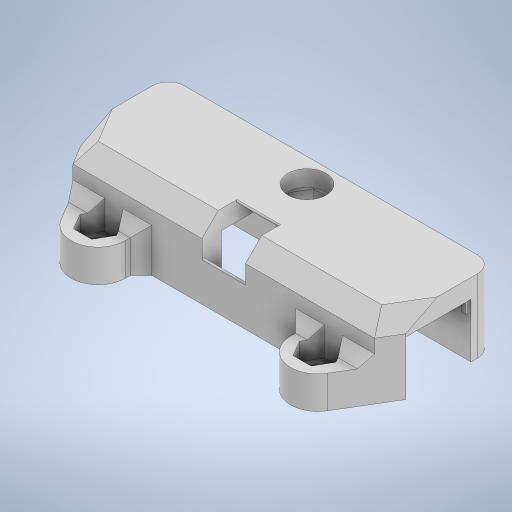
# Autodesk Inventor part: uchwyt_silnikow
Saved by Autodesk Inventor 2023 (Build 270158000, 158)
## iProperties
Created: 2023-08-17
Part Number: uchwyt_silnikow
Material: Ogólny
Document SubType Name: Modeling
Designer: Kamil
Density: 1 g/cm^3
Appearance: Domyślna
Author: Kamil
Autodesk Inventor part; units mm, degrees
ref_plane "YZ Plane" through (0, 0, 0) normal (1, 0, 0) x (0, 1, 0)
ref_plane "XZ Plane" through (0, 0, 0) normal (0, 1, 0) x (-1, 0, 0)
ref_plane "XY Plane" through (0, 0, 0) normal (0, 0, 1) x (1, 0, 0)
sketch "Szkic1" plane through (0, 0, 0) normal (0, 1, 0) x (-1, 0, 0)
  circle A0 centre (-9.75, 6.5) radius 1.75
  circle A1 centre (-50.25, 6.5) radius 1.75
  arc A2 (-31.4825, -12) -> (-28.5175, -12) centre (-30, -11.7713) ccw
  arc A3 (-28.5175, -12) -> (-31.4825, -12) centre (-30, -11.7713) ccw
  arc A4 (-3, -16.2) -> (0, -13.2) centre (-3, -13.2) ccw
  line L0 (0, -12) -> (0, -13.2)
  line L1 (-25.5772, -12) -> (0, -12)
  line L2 (-28.5175, -12) -> (-25.5772, -12)
  arc A5 (-31.4825, -12) -> (-28.5175, -12) centre (-30, -11.7713) ccw
  line L3 (-31.4825, -12) -> (-34.4228, -12)
  line L4 (-34.4228, -12) -> (-60, -12)
  line L5 (-60, -12) -> (-60, -13.2)
  arc A6 (-60, -13.2) -> (-57, -16.2) centre (-57, -13.2) ccw
  line L6 (-3, -16.2) -> (-57, -16.2)
  circle A7 centre (-50.25, 6.5) radius 1.75
  line L7 (-24.852, 0) -> (0, 0)
  line L8 (-35.148, 0) -> (-60, 0)
  circle A8 centre (-9.75, 6.5) radius 1.75
  circle A9 centre (-50.25, 6.5) radius 5
  circle A10 centre (-9.75, 6.5) radius 5
  line L9 (-60, 0) -> (-54.5335, 9.0791)
  line L10 (0, 0) -> (-5.4665, 9.0791)
  line L11 (-14.75, 6.5) -> (-14.75, 0)
  line L12 (-45.25, 6.5) -> (-45.25, 0)
  arc A11 (-27.6792, -16.2) -> (-32.3208, -16.2) centre (-30, -11.7713) ccw
  point P0 (-25.0052, -12)
  point P1 (-34.9948, -12)
  dimension "d0" = 10
  dimension "d1" = 10
  dimension "d2" = 10
  constraints: 26 end point, 16 point on circle, 12 centre point, 6 horizontal, 4 point on line, 4 tangent, 3 coincident, 1 perpendicular, 1 vertical, 4 other
  measures "d0" diameter of A9
  measures "d1" diameter of A10
  measures "d2" diameter of A11
extrude "Wyciągnięcie proste1" add sketch "Szkic1" along normal blind 10 contours L3 L4 A11 L1 L2 A3 | A2 L2 L1 A11 L6 L4 L3 | A11 L6 A6 L5 L4 | L1 L0 A4 L6 A11 | L11 A10 L10 L7 | A10 | L8 L9 A9 L12 | A9
sketch "Szkic2" plane through (0, 10, 0) normal (0, 1, 0) x (1, 0, 0)
  line L0 (57, 16.2) -> (3, 16.2) projected
  arc A0 (3, 16.2) -> (0, 13.2) centre (3, 13.2) ccw projected
  line L1 (0, 13.2) -> (0, 12) projected
  line L2 (0, 12) -> (25.0052, 12) projected
  arc A1 (25.0052, 12) -> (34.9948, 12) centre (30, 11.7713) ccw projected
  line L3 (34.9948, 12) -> (60, 12) projected
  line L4 (60, 12) -> (60, 13.2) projected
  arc A2 (60, 13.2) -> (57, 16.2) centre (57, 13.2) ccw projected
  circle A3 centre (30, 11.7713) radius 1.5 projected
  line L5 (14.75, 0) -> (0, 0) projected
  line L6 (0, 0) -> (5.4665, -9.0791) projected
  arc A4 (5.4665, -9.0791) -> (14.75, -6.5) centre (9.75, -6.5) ccw projected
  line L7 (14.75, -6.5) -> (14.75, 0) projected
  circle A5 centre (9.75, -6.5) radius 1.75 projected
  arc A6 (45.25, -6.5) -> (54.5335, -9.0791) centre (50.25, -6.5) ccw projected
  line L8 (54.5335, -9.0791) -> (60, 0) projected
  line L9 (60, 0) -> (45.25, 0) projected
  line L10 (45.25, 0) -> (45.25, -6.5) projected
  circle A7 centre (50.25, -6.5) radius 1.75 projected
  line L11 (0, 0) -> (60, 0)
  line L12 (60, 0) -> (60, 12)
  line L13 (60, 12) -> (0, 12)
  line L14 (0, 12) -> (0, 0)
  constraints: 8 end point, 2 parallel, 1 horizontal, 1 perpendicular
extrude "Wyciągnięcie proste2" add sketch "Szkic2" along normal blind 3.5 contours A2 L4 L3 L13 A3 L2 L1 A0 L0 | L12 L9 L11 L5 L14 L2 A1 L3 | A1 L13 A3 | L8 A6 L10 L9 | L5 L7 A4 L6
sketch "Szkic3" plane through (0, 0, 0) normal (0, -1, 0) x (1, 0, 0)
  line L0 (14.75, 0) -> (0, 0) projected
  line L1 (14.75, 6.5) -> (14.75, 0) projected
  arc A0 (14.75, 6.5) -> (5.4665, 9.0791) centre (9.75, 6.5) ccw projected
  line L2 (0, 0) -> (5.4665, 9.0791) projected
  circle A1 centre (9.75, 6.5) radius 1.75 projected
  arc A2 (54.5335, 9.0791) -> (45.25, 6.5) centre (50.25, 6.5) ccw projected
  line L3 (45.25, 0) -> (45.25, 6.5) projected
  line L4 (60, 0) -> (45.25, 0) projected
  line L5 (54.5335, 9.0791) -> (60, 0) projected
  circle A3 centre (50.25, 6.5) radius 1.75 projected
  line L6 (14.75, 0) -> (45.25, 0) projected
  line L7 (45.25, 0) -> (14.75, 0)
  line L8 (14.75, 0) -> (14.75, 4)
  line L9 (14.75, 4) -> (45.25, 4)
  line L10 (45.25, 4) -> (45.25, 0)
  dimension "d7" = 4
  constraints: 8 end point, 2 parallel, 1 horizontal, 1 perpendicular, 1 point on line
  measures "d7" distance of L7.end L8.end
extrude "Wyciągnięcie proste3" add sketch "Szkic3" against normal up to surface (13.5 mm away) contours L1 L9 L3 L6
sketch "Szkic4" plane through (0, 13.5, 0) normal (0, 1, 0) x (1, 0, 0)
  circle A0 centre (9.75, -6.5) radius 1.75 projected
  circle A1 centre (50.25, -6.5) radius 1.75 projected
  circle A2 centre (9.75, -6.5) radius 2.9
  circle A3 centre (50.25, -6.5) radius 2.9
  line L0 (11.4243, -3.6) -> (13.0986, -6.5)
  line L1 (13.0986, -6.5) -> (11.4243, -9.4)
  line L2 (11.4243, -9.4) -> (8.0757, -9.4)
  line L3 (8.0757, -9.4) -> (6.4014, -6.5)
  line L4 (6.4014, -6.5) -> (8.0757, -3.6)
  line L5 (8.0757, -3.6) -> (11.4243, -3.6)
  line L6 (51.9243, -3.6) -> (53.5986, -6.5)
  line L7 (53.5986, -6.5) -> (51.9243, -9.4)
  line L8 (51.9243, -9.4) -> (48.5757, -9.4)
  line L9 (48.5757, -9.4) -> (46.9014, -6.5)
  line L10 (46.9014, -6.5) -> (48.5757, -3.6)
  line L11 (48.5757, -3.6) -> (51.9243, -3.6)
  line L12 (0, 0) -> (5.4665, -9.0791) projected
  line L13 (2.1676, -3.6) -> (57.8324, -3.6)
  line L14 (54.5335, -9.0791) -> (60, 0) projected
  arc A4 (60, 13.2) -> (57, 16.2) centre (57, 13.2) ccw projected
  line L15 (57, 16.2) -> (3, 16.2) projected
  arc A5 (3, 16.2) -> (0, 13.2) centre (3, 13.2) ccw projected
  line L16 (0, 13.2) -> (0, 0) projected
  line L17 (0, 0) -> (5.4665, -9.0791) projected
  arc A6 (5.4665, -9.0791) -> (14.75, -6.5) centre (9.75, -6.5) ccw projected
  line L18 (14.75, -6.5) -> (14.75, -4) projected
  line L19 (45.25, -4) -> (14.75, -4) projected
  line L20 (45.25, -4) -> (45.25, -6.5) projected
  arc A7 (45.25, -6.5) -> (54.5335, -9.0791) centre (50.25, -6.5) ccw projected
  line L21 (54.5335, -9.0791) -> (60, 0) projected
  line L22 (60, 0) -> (60, 13.2) projected
  circle A8 centre (9.75, -6.5) radius 1.75 projected
  circle A9 centre (50.25, -6.5) radius 1.75 projected
  circle A10 centre (30, 11.7713) radius 1.5 projected
  point P0 (9.75, -3.6)
  point P1 (50.25, -3.6)
  dimension "d10" = 5.8
  dimension "d11" = 5.8
  constraints: 26 end point, 4 coincident, 3 point on line, 2 midpoint, 2 vertical alignment, 1 horizontal, 30 other
extrude "Wyciągnięcie proste4" cut sketch "Szkic4" against normal blind 7.5 contours L0 L13 L10 L9 L8 L7 L6 L14 A7 L20 L19 L18 A6 L12 L4 L3 L2 L1
extrude "Wyciągnięcie proste5" cut sketch "Szkic4" against normal blind 10.8 contours A0 | A1 | A2 | A2 L0 L1 | A2 L5 L0 | L1 L2 A2 | A2 L4 L5 | L2 L3 A2 | A2 L3 L4 | L11 A3 L10 | A3 | A3 L9 L10 | L11 L6 A3 | A3 L8 L9 | L6 L7 A3 | A3 L7 L8
sketch "Szkic5" plane through (0, 6, 0) normal (0, 1, 0) x (1, 0, 0)
  line L0 (14.75, -4) -> (14.75, -6.5) projected
  line L1 (45.25, -4) -> (14.75, -4) projected
  line L2 (45.25, -6.5) -> (45.25, -4) projected
  arc A0 (45.25, -6.5) -> (54.5335, -9.0791) centre (50.25, -6.5) ccw projected
  line L3 (57.8324, -3.6) -> (54.5335, -9.0791) projected
  line L4 (51.9243, -3.6) -> (57.8324, -3.6) projected
  line L5 (53.5986, -6.5) -> (51.9243, -3.6) projected
  line L6 (51.9243, -9.4) -> (53.5986, -6.5) projected
  line L7 (48.5757, -9.4) -> (51.9243, -9.4) projected
  line L8 (46.9014, -6.5) -> (48.5757, -9.4) projected
  line L9 (48.5757, -3.6) -> (46.9014, -6.5) projected
  line L10 (11.4243, -3.6) -> (48.5757, -3.6) projected
  line L11 (13.0986, -6.5) -> (11.4243, -3.6) projected
  line L12 (11.4243, -9.4) -> (13.0986, -6.5) projected
  line L13 (8.0757, -9.4) -> (11.4243, -9.4) projected
  line L14 (6.4014, -6.5) -> (8.0757, -9.4) projected
  line L15 (8.0757, -3.6) -> (6.4014, -6.5) projected
  line L16 (2.1676, -3.6) -> (8.0757, -3.6) projected
  line L17 (5.4665, -9.0791) -> (2.1676, -3.6) projected
  arc A1 (5.4665, -9.0791) -> (14.75, -6.5) centre (9.75, -6.5) ccw projected
  line L18 (14.75, -4) -> (14.75, -3.6)
  line L19 (45.25, -4) -> (45.25, -3.6)
  point P0 (0, 0)
  constraints: 4 end point, 2 perpendicular, 2 point on line
extrude "Wyciągnięcie proste6" cut sketch "Szkic5" against normal through all contours L18 L10 L19 L1
sketch "Szkic6" plane through (0, 13.5, 0) normal (0, 1, 0) x (1, 0, 0)
  circle A0 centre (30, 11.7713) radius 1.5 projected
  circle A1 centre (30, 11.7713) radius 2.9
  circle A2 centre (30, 11.7713) radius 1.5 projected
  line L0 (31.6743, 14.6713) -> (33.3486, 11.7713)
  line L1 (33.3486, 11.7713) -> (31.6743, 8.8713)
  line L2 (31.6743, 8.8713) -> (28.3257, 8.8713)
  line L3 (28.3257, 8.8713) -> (26.6514, 11.7713)
  line L4 (26.6514, 11.7713) -> (28.3257, 14.6713)
  line L5 (28.3257, 14.6713) -> (31.6743, 14.6713)
  circle A3 centre (30, 11.7713) radius 3.5
  point P0 (0, 0)
  point P1 (30, 14.6713)
  dimension "d20" = 5.8
  dimension "d21" = 7
  constraints: 12 end point, 3 coincident, 1 centre point, 1 midpoint, 1 vertical alignment, 15 other
  measures "d21" diameter of A3
extrude "Wyciągnięcie proste7" cut sketch "Szkic6" against normal blind 3 contours A0 | A1 | A1 L0 L1 | A1 L5 L0 | L1 L2 A1 | A1 L4 L5 | L2 L3 A1 | A1 L3 L4 | A3
extrude "Wyciągnięcie proste8" cut sketch "Szkic6" against normal blind 6 contours A0 | A1 | A1 L0 L1 | A1 L5 L0 | L1 L2 A1 | A1 L4 L5 | L2 L3 A1 | A1 L3 L4
sketch "Szkic7" plane through (0, 10, 0) normal (0, -1, 0) x (1, 0, 0)
  line L0 (60, 0) -> (0, 0) projected
  line L1 (0, -12) -> (0, 0) projected
  line L2 (0, -12) -> (25.0052, -12) projected
  arc A0 (34.9948, -12) -> (25.0052, -12) centre (30, -11.7713) ccw projected
  line L3 (34.9948, -12) -> (60, -12) projected
  line L4 (60, 0) -> (60, -12) projected
  line L5 (34.9948, -12) -> (60, -12) projected
  line L6 (59.4, -12) -> (58.7, -12)
  line L7 (58.7, -12) -> (58.7, -9)
  line L8 (58.7, -9) -> (59.4, -9)
  line L9 (59.4, -9) -> (59.4, -12)
  line L10 (53.6, -12) -> (51.6, -12)
  line L11 (51.6, -12) -> (51.6, -9)
  line L12 (51.6, -9) -> (53.6, -9)
  line L13 (53.6, -9) -> (53.6, -12)
  circle A1 centre (30, -11.7713) radius 1.5 projected
  line L14 (30, -11.7713) -> (30, 0)
  line L15 (60, 0) -> (0, 0) projected
  line L16 (1.3, -12) -> (1.3, -9)
  line L17 (1.3, -9) -> (0.6, -9)
  line L18 (0.6, -9) -> (0.6, -12)
  line L19 (8.4, -12) -> (8.4, -9)
  line L20 (8.4, -9) -> (6.4, -9)
  line L21 (6.4, -9) -> (6.4, -12)
  point P0 (58.7, -10.5)
  point P1 (53.6, -10.5)
  dimension "d26" = 0.7
  dimension "d27" = 3
  dimension "d28" = 0.6
  dimension "d29" = 2
  dimension "d30" = 5.1
  dimension "d31" = 3
  constraints: 30 end point, 8 symmetric about line, 4 parallel, 3 midpoint, 2 horizontal, 2 perpendicular, 2 point on line
  measures "d26" distance of L7.end L8.end
  measures "d27" distance of L6.end L7.end
  measures "d28" distance between parallel lines of L4 L9
  measures "d29" distance of L11.end L12.end
  measures "d30" distance of point (58.7, -10.5) point (53.6, -10.5)
  measures "d31" distance of L10.end L11.end
extrude "Wyciągnięcie proste9" add sketch "Szkic7" along normal blind 0.4 contours L3 L7 L8 L9 | L18 L17 L16 L2 | L11 L12 L13 L3 | L2 L21 L20 L19
sketch "Szkic8" plane through (34.9948, 0, -12) normal (0, 0, 1) x (1, 0, 0)
  line L0 (-33.6948, 9.6) -> (-34.3948, 9.6) projected
  line L1 (-26.5948, 9.6) -> (-28.5948, 9.6) projected
  line L2 (18.6052, 9.6) -> (16.6052, 9.6) projected
  line L3 (24.4052, 9.6) -> (23.7052, 9.6) projected
  line L4 (-34.3948, 9.6) -> (-34.3948, 10) projected
  line L5 (-34.3948, 9.6) -> (-33.6948, 9.6)
  line L6 (-33.6948, 9.6) -> (-33.6948, 7.5)
  line L7 (-33.6948, 7.5) -> (-34.3948, 7.5)
  line L8 (-34.3948, 7.5) -> (-34.3948, 9.6)
  line L9 (-26.5948, 9.6) -> (-28.5948, 9.6)
  line L10 (-28.5948, 9.6) -> (-28.5948, 7.5)
  line L11 (-28.5948, 7.5) -> (-26.5948, 7.5)
  line L12 (-26.5948, 7.5) -> (-26.5948, 9.6)
  line L13 (24.4052, 9.6) -> (23.7052, 9.6)
  line L14 (23.7052, 9.6) -> (23.7052, 7.5)
  line L15 (23.7052, 7.5) -> (24.4052, 7.5)
  line L16 (24.4052, 7.5) -> (24.4052, 9.6)
  line L17 (18.6052, 9.6) -> (16.6052, 9.6)
  line L18 (16.6052, 9.6) -> (16.6052, 7.5)
  line L19 (16.6052, 7.5) -> (18.6052, 7.5)
  line L20 (18.6052, 7.5) -> (18.6052, 9.6)
  point P0 (-34.9948, 0)
  dimension "d34" = 2.1
  dimension "d35" = 2.1
  dimension "d36" = 2.1
  dimension "d37" = 2.1
  constraints: 32 end point, 8 parallel, 4 horizontal, 4 perpendicular
  measures "d34" distance of L5.end L6.end
  measures "d35" distance of L10.end L9.end
  measures "d36" distance of L14.end L13.end
  measures "d37" distance of L18.end L17.end
extrude "Wyciągnięcie proste10" add sketch "Szkic8" along normal blind 0.4
sketch "Szkic10" plane through (0, 13.5, 0) normal (0, 1, 0) x (1, 0, 0)
  line L0 (2.1676, -3.6) -> (57.8324, -3.6) projected
  line L1 (30, -3.6) -> (34, -3.6)
  line L2 (34, -3.6) -> (34, 2.4)
  line L3 (34, 2.4) -> (30, 2.4)
  line L4 (30, 2.4) -> (30, -3.6)
  line L5 (30, 2.4) -> (26, 2.4)
  line L6 (26, 2.4) -> (26, -3.6)
  line L7 (26, -3.6) -> (30, -3.6)
  line L8 (30, -3.6) -> (30, 2.4)
  point P0 (0, 0)
  dimension "d44" = 4
  dimension "d45" = 6
  constraints: 16 end point, 4 parallel, 2 horizontal, 2 perpendicular, 1 midpoint, 1 point on line
  measures "d44" distance of L3.end L2.end
  measures "d45" distance of L2.end L1.end
extrude "Wyciągnięcie proste12" cut sketch "Szkic10" against normal blind 6
chamfer "Faza1" distance 3.5 angle 45 2 edges at (30, 10, -2.4) (30, 7.5, 0)
fillet "Zaokrąglenie3" radius 0.2 2 edges at (30, 7.5, 3.4999) (30, 7.5, 3.6)
fillet "Zaokrąglenie4" radius 0.2 4 edges at (34, 13.5, -2.4) (30, 13.4999, -2.4) (30, 13.5, -2.4) (26, 13.5, -2.4)
chamfer "Faza2" distance 3 angle 45 4 edges at (1.0838, 13.5, 1.8) (14.0838, 13.5, 3.6) (45.9162, 13.5, 3.6) (58.9162, 13.5, 1.8)
chamfer "Faza3" distance 2 angle 45 6 edges at (13.0872, 6, 3.6) (5.1216, 6, 3.6) (46.9128, 6, 3.6) (54.8784, 6, 3.6) (45.25, 3, 3.6) (14.75, 3, 3.6)
sketch "Szkic11" plane through (0, 0, 0) normal (0, -1, 0) x (1, 0, 0)
  circle A0 centre (30, -11.7713) radius 1.5 projected
  circle A1 centre (30, -11.7713) radius 4.1262
  line L0 (57, -16.2) -> (3, -16.2) projected
  arc A2 (57, -16.2) -> (60, -13.2) centre (57, -13.2) ccw projected
  line L1 (60, -12) -> (60, -13.2) projected
  line L2 (34.9948, -12) -> (60, -12) projected
  arc A3 (34.9948, -12) -> (25.0052, -12) centre (30, -11.7713) ccw projected
  line L3 (0, -12) -> (25.0052, -12) projected
  line L4 (0, -13.2) -> (0, -12) projected
  arc A4 (0, -13.2) -> (3, -16.2) centre (3, -13.2) ccw projected
  circle A5 centre (30, -11.7713) radius 1.5 projected
  line L5 (25.0052, -12) -> (25.8801, -12)
  line L6 (34.9948, -12) -> (51.6, -12) projected
  line L7 (34.9948, -12) -> (34.1199, -12)
  point P0 (0, 0)
  constraints: 4 end point, 2 point on circle, 1 centre point, 1 coincident, 1 horizontal, 1 point on line
extrude "Wyciągnięcie proste13" cut sketch "Szkic11" against normal up to surface (10 mm away) contours A1 L5 A3 L7
